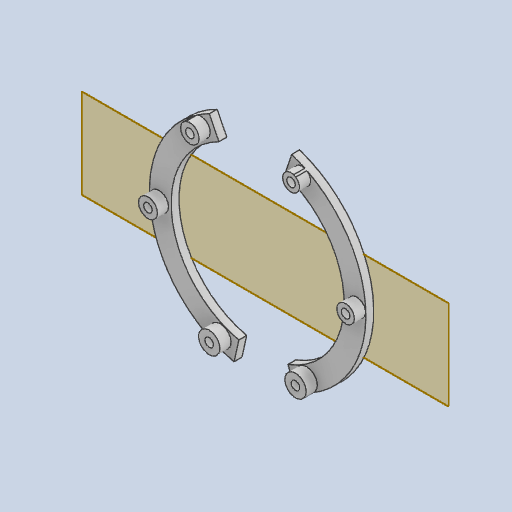
# Autodesk Inventor part: Part5
Saved by Autodesk Inventor 2023.1 (Build 271208000, 208)
## iProperties
Created: 2022-12-26
Part Number: Part5
Material: Generic
Document SubType Name: Modeling
Designer: USER
Density: 1 g/cm^3
Appearance: Default
Author: USER
## iProperties of the stored document Part5_3DPrint.ipt
Created: 2022-12-26
Part Number: Part5_3DPrint
Material: Generic
Document SubType Name: Modeling
Designer: USER
Density: 1 g/cm^3
Appearance: Default
Author: USER
Autodesk Inventor part; units mm, degrees
ref_plane "YZ Plane" through (0, 0, 0) normal (1, 0, 0) x (0, 1, 0)
ref_plane "XZ Plane" through (0, 0, 0) normal (0, 1, 0) x (-1, 0, 0)
ref_plane "XY Plane" through (0, 0, 0) normal (0, 0, 1) x (1, 0, 0)
ref_plane "Work Plane1" through (0, 0, 0.254) normal (0, 0, 1) x (1, 0, 0)
sketch "Sketch1" plane through (0, 0, 0.254) normal (0, 0, 1) x (1, 0, 0)
  line L0 (-30.3342, -3.8452) -> (-34.0294, 3.542) projected
  arc A0 (-34.0294, 3.542) -> (-24.5515, -73.6045) centre (-15.5698, -33.3456) ccw projected
  line L1 (-24.5515, -73.6045) -> (-22.7534, -65.536) projected
  arc A1 (-32.8607, -61.4358) -> (-22.7534, -65.536) centre (-15.579, -33.3432) ccw projected
  arc A2 (-48.0416, -39.1767) -> (-32.8607, -61.4358) centre (-15.579, -33.3432) ccw projected
  arc A3 (-48.3364, -29.496) -> (-48.0416, -39.1767) centre (-15.579, -33.3432) ccw projected
  arc A4 (-38.6838, -9.8057) -> (-48.3364, -29.496) centre (-15.579, -33.3432) ccw projected
  arc A5 (-30.3342, -3.8452) -> (-38.6838, -9.8057) centre (-15.579, -33.3432) ccw projected
  circle A6 centre (-37.1718, -2.3566) radius 1.65 projected
  circle A7 centre (-53.1457, -34.9208) radius 1.65 projected
  circle A8 centre (-29.7865, -67.7339) radius 1.65 projected
  line L2 (-4.0023, -64.2273) -> (-1.099, -71.9726) projected
  arc A9 (-1.099, -71.9726) -> (-2.6102, 5.8143) centre (-15.5698, -33.3456) ccw projected
  line L3 (-2.6102, 5.8143) -> (-5.2093, -2.0332) projected
  arc A10 (3.0091, -6.0975) -> (-5.2093, -2.0332) centre (-15.579, -33.3432) ccw projected
  arc A11 (16.7844, -26.9826) -> (3.0091, -6.0975) centre (-15.579, -33.3432) ccw projected
  arc A12 (17.1784, -37.1904) -> (16.7844, -26.9826) centre (-15.579, -33.3432) ccw projected
  arc A13 (4.9019, -59.1962) -> (17.1784, -37.1904) centre (-15.579, -33.3432) ccw projected
  arc A14 (-4.0023, -64.2273) -> (4.9019, -59.1962) centre (-15.579, -33.3432) ccw projected
  circle A15 centre (1.4037, 0.7229) radius 1.65 projected
  circle A16 centre (22.2051, -32.2206) radius 1.65 projected
  circle A17 centre (3.1034, -65.5014) radius 1.65 projected
  circle A18 centre (-53.1457, -34.9208) radius 3.5999
  circle A19 centre (-37.1718, -2.3566) radius 3.5122
  circle A20 centre (1.4037, 0.7229) radius 3.2143
  circle A21 centre (22.2051, -32.2206) radius 3.3528
  circle A22 centre (3.1034, -65.5014) radius 4.076
  circle A23 centre (-29.7865, -67.7339) radius 4.0534
  point P0 (0, 0)
  point P1 (2.4269, 3.77)
  point P2 (3.22, 3.3748)
  point P3 (5.4258, -68.851)
  point P4 (4.8616, -69.1787)
  point P5 (-30.9787, -71.6081)
  point P6 (-31.6782, -71.3189)
  point P7 (-39.602, 0.179)
  point P8 (-38.7101, 0.8007)
  constraints: 6 centre point, 6 coincident
extrude "Extrusion1" add sketch "Sketch1" along normal blind 7 contours A19 A0 | A23 A0 | A22 A9 | A20 A9 | A18 | A21 picked at (-34.3318, -2.7742) picked at (-26.5918, -67.2698) picked at (6.314, -65.0394) picked at (4.0492, 1.1119)
ref_plane "Work Plane2" through (0, 0, 0) normal (0, 0, 1) x (1, 0, 0)
sketch "Sketch2" plane through (0, 0, 0) normal (0, 0, 1) x (1, 0, 0)
  line L0 (-30.3342, -3.8452) -> (-34.0294, 3.542) projected
  arc A0 (-34.0294, 3.542) -> (-24.5515, -73.6045) centre (-15.5698, -33.3456) ccw projected
  line L1 (-24.5515, -73.6045) -> (-22.7534, -65.536) projected
  arc A1 (-32.8607, -61.4358) -> (-22.7534, -65.536) centre (-15.579, -33.3432) ccw projected
  arc A2 (-48.0416, -39.1767) -> (-32.8607, -61.4358) centre (-15.579, -33.3432) ccw projected
  arc A3 (-48.3364, -29.496) -> (-48.0416, -39.1767) centre (-15.579, -33.3432) ccw projected
  arc A4 (-38.6838, -9.8057) -> (-48.3364, -29.496) centre (-15.579, -33.3432) ccw projected
  arc A5 (-30.3342, -3.8452) -> (-38.6838, -9.8057) centre (-15.579, -33.3432) ccw projected
  circle A6 centre (-37.1718, -2.3566) radius 1.65 projected
  circle A7 centre (-53.1457, -34.9208) radius 1.65 projected
  circle A8 centre (-29.7865, -67.7339) radius 1.65 projected
  line L2 (-4.0023, -64.2273) -> (-1.099, -71.9726) projected
  arc A9 (-1.099, -71.9726) -> (-2.6102, 5.8143) centre (-15.5698, -33.3456) ccw projected
  line L3 (-2.6102, 5.8143) -> (-5.2093, -2.0332) projected
  arc A10 (3.0091, -6.0975) -> (-5.2093, -2.0332) centre (-15.579, -33.3432) ccw projected
  arc A11 (16.7844, -26.9826) -> (3.0091, -6.0975) centre (-15.579, -33.3432) ccw projected
  arc A12 (17.1784, -37.1904) -> (16.7844, -26.9826) centre (-15.579, -33.3432) ccw projected
  arc A13 (4.9019, -59.1962) -> (17.1784, -37.1904) centre (-15.579, -33.3432) ccw projected
  arc A14 (-4.0023, -64.2273) -> (4.9019, -59.1962) centre (-15.579, -33.3432) ccw projected
  circle A15 centre (1.4037, 0.7229) radius 1.65 projected
  circle A16 centre (22.2051, -32.2206) radius 1.65 projected
  circle A17 centre (3.1034, -65.5014) radius 1.65 projected
  point P0 (0, 0)
extrude "Extrusion2" add sketch "Sketch2" along normal blind 3
body "Solid1"
